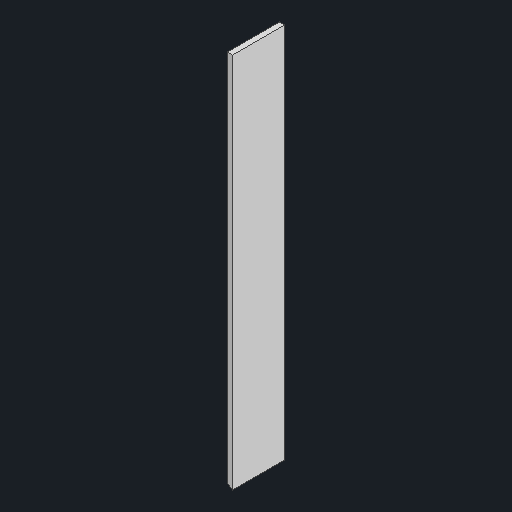
# Autodesk Inventor part: DMF 01 53 side part v2.1
Saved by Autodesk Inventor 2026.2 (Build 302298010, 298A)
## iProperties
Created: 2024-05-05
Part Number: DMF 01 53 side part v2.1
Material: Generic
Document SubType Name: Modeling
Designer: pokla
Density: 1 g/cm^3
Appearance: Default
Author: pokla
Autodesk Inventor part; units mm, degrees
ref_plane "YZ Plane" through (0, 0, 0) normal (1, 0, 0) x (0, 1, 0)
ref_plane "XZ Plane" through (0, 0, 0) normal (0, 1, 0) x (-1, 0, 0)
ref_plane "XY Plane" through (0, 0, 0) normal (0, 0, 1) x (1, 0, 0)
sketch "Sketch1" plane through (0, 0, 0) normal (0, 0, 1) x (1, 0, 0)
  line L0 (0, 286.8339) -> (202.8222, 202.8222) construction
  line L1 (202.8222, 202.8222) -> (286.8339, 0) construction
  line L2 (286.8339, 0) -> (202.8222, -202.8222) construction
  line L3 (202.8222, -202.8222) -> (0, -286.8339) construction
  line L4 (0, -286.8339) -> (-202.8222, -202.8222) construction
  line L5 (-202.8222, -202.8222) -> (-286.8339, 0) construction
  line L6 (-286.8339, 0) -> (-202.8222, 202.8222) construction
  line L7 (-202.8222, 202.8222) -> (0, 286.8339) construction
  line L8 (-202.8222, 202.8222) -> (0, 286.8339) construction
  line L9 (-464.5194, 781.7427) -> (-224.3107, 881.2404) construction
  line L10 (-101.4111, 244.8281) -> (-344.4151, 831.4916) construction
  line L11 (-224.3107, 881.2404) -> (0, 881.2404) construction
  line L12 (0, 881.2404) -> (0, 286.8339) construction
  line L13 (-464.5194, 781.7427) -> (-623.1311, 623.1311) construction
  line L14 (-623.1311, 623.1311) -> (-202.8222, 202.8222) construction
  line L15 (-5, 290.1748) -> (-201.6491, 208.7201) construction
  line L16 (-201.6491, 208.7201) -> (-616.06, 623.1311) construction
  line L17 (-616.06, 623.1311) -> (-461.6872, 777.5039) construction
  line L18 (-461.6872, 777.5039) -> (-223.3162, 876.2404) construction
  line L19 (-223.3162, 876.2404) -> (-5, 876.2404) construction
  line L20 (-5, 876.2404) -> (-5, 290.1748) construction
  line L21 (-13, 295.5203) -> (-199.772, 218.1568) construction
  line L22 (-199.772, 218.1568) -> (-604.7463, 623.1311) construction
  line L23 (-604.7463, 623.1311) -> (-457.1555, 770.7219) construction
  line L24 (-457.1555, 770.7219) -> (-221.7249, 868.2404) construction
  line L25 (-221.7249, 868.2404) -> (-13, 868.2404) construction
  line L26 (-13, 868.2404) -> (-13, 295.5203) construction
  line L27 (-13, 868.2404) -> (-5, 868.2404)
  line L28 (-5, 868.2404) -> (-5, 290.1748)
  line L29 (-5, 290.1748) -> (-13, 295.5203)
  line L30 (-13, 295.5203) -> (-13, 868.2404)
  point P0 (0, 0)
  point P1 (0, 0)
  point P2 (0, 0)
  dimension "d0" = 530
  dimension "d1" = 260
  dimension "d2" = 635
  dimension "d10" = 5
  dimension "d11" = 8
  constraints: 62 end point, 3 perpendicular, 2 coincident, 2 midpoint, 1 collinear, 1 horizontal, 1 parallel, 1 point on line, 1 symmetric about line, 1 vertical, 1 vertical alignment, 27 other
  measures "d0" distance between parallel lines of L5 L1
  measures "d1" distance of L13.start L11.start
  measures "d2" distance of L10.end L10.start
  measures "d10" distance between parallel lines of L12 L20
  measures "d11" distance between parallel lines of L20 L26
extrude "Extrusion1" add sketch "Sketch1" against normal blind 80
equation "\"d0\" = Барабан_размер_по_плоскостям"
equation "\"d1\" = Кассета_длина_грани"
equation "\"d2\" = Кассета_высота"
equation "\"Барабан_размер_по_плоскостям\" = 530"
equation "\"Кассета_длина_грани\" = 260"
equation "\"Кассета_высота\" = 635"
body "Solid1"
